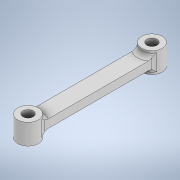
# Autodesk Inventor part: connecting rod
Saved by Autodesk Inventor 2020 (Build 240168000, 168)
## iProperties
Created: 2020-08-08
Part Number: connecting rod
Material: Generic
Document SubType Name: Modeling
Designer: benny
Density: 1 g/cm^3
Appearance: Default
Author: benny
Autodesk Inventor part; units mm, degrees
ref_plane "YZ Plane" through (0, 0, 0) normal (1, 0, 0) x (0, 1, 0)
ref_plane "XZ Plane" through (0, 0, 0) normal (0, 1, 0) x (-1, 0, 0)
ref_plane "XY Plane" through (0, 0, 0) normal (0, 0, 1) x (1, 0, 0)
sketch "Sketch1" plane through (0, 0, 0) normal (0, 1, 0) x (-1, 0, 0)
  line L0 (-4, 27) -> (-4, -27)
  line L1 (-4, -30) -> (-2.5, -30)
  line L2 (4, -27) -> (4, 27)
  line L3 (4, 30) -> (-4, -30) construction
  line L4 (-3.5275, 26.4565) -> (4, -30) construction
  circle A0 centre (0, 30) radius 5
  circle A1 centre (0, -30) radius 5
  circle A2 centre (0, 30) radius 2.5
  circle A3 centre (0, -30) radius 2.5
  line L5 (-2.5, 30) -> (-4, 30)
  point P0 (0, 0)
  dimension "d4" = 5
  dimension "d5" = 5
  dimension "d0" = 8
  dimension "d1" = 60
  dimension "d2" = 10
  dimension "d3" = 10
  constraints: 12 end point, 5 point on circle, 2 centre point, 2 coincident, 2 horizontal alignment, 2 parallel, 2 point on line, 1 horizontal, 1 midpoint, 1 perpendicular, 4 other
  measures "d0" distance of L4.end L1.start
  measures "d1" distance of L1.start L5.end
  measures "d2" diameter of A0
  measures "d3" diameter of A1
extrude "Extrusion1" add sketch "Sketch1" along normal mid plane 4
sketch "Sketch3" plane through (0, 2, 0) normal (0, 1, 0) x (1, 0, 0)
  arc A0 (-4, -27) -> (4, -27) centre (0, -30) ccw projected
  circle A1 centre (0, -30) radius 5
  circle A2 centre (0, -30) radius 2.5
  circle A3 centre (0, 30) radius 2.5 projected
  circle A4 centre (0, 30) radius 5
  circle A5 centre (0, 30) radius 2.5
  point P0 (0, 0)
  point P1 (4, -27)
  dimension "d8" = 10
  dimension "d9" = 5
  constraints: 4 centre point, 4 coincident
  measures "d8" diameter of A4
  measures "d9" diameter of A5
extrude "Extrusion2" add sketch "Sketch3" along normal blind 3
fillet "Fillet1" radius 2 2 edges at (0, 2, 25) (0, 2, -25)
fillet "Fillet2" radius 4 5 edges at (4, 1, 27) (4, 3, -27) (4, 0, -27) (-4, 1, 27) (-4, 1, -27)
mirror "Mirror1" about plane through (0, 0, 0) normal (0, 1, 0) of "Extrusion2"
fillet "Fillet3" radius 2 3 edges at (4.2371, -2, 27.3454) (-0.4186, -2, 25.0175) (0, -2, -25)
body "Solid1"
